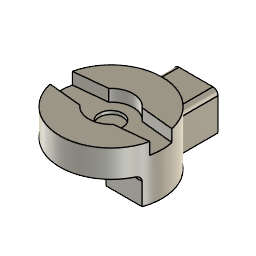
valve_coupler (Autodesk Fusion 360 design; units mm, degrees)
Autodesk Fusion 360 part; units mm, degrees
sketch "Sketch1" plane through (0, 0, 0) normal (0, 0, 1) x (1, 0, 0)
  circle A0 centre (0, 0) radius 6.5
  line L0 (-15, 0) -> (15, 0) construction
  line L1 (0, 15) -> (0, -15) construction
  arc A1 (-14.6437, -3.25) -> (0, -15) centre (0, 0) ccw
  arc A2 (14.6437, -3.25) -> (14.6437, 3.25) centre (0, 0) ccw
  arc A3 (-14.6437, 3.25) -> (-14.6437, -3.25) centre (0, 0) ccw
  arc A4 (0, 15) -> (-14.6437, 3.25) centre (0, 0) ccw
  arc A5 (0, -15) -> (14.6437, -3.25) centre (0, 0) ccw
  arc A6 (14.6437, 3.25) -> (0, 15) centre (0, 0) ccw
  line L2 (4.9181, 4.25) -> (4.9181, -4.25)
  line L3 (14.6437, 3.25) -> (14.6437, -3.25)
  line L4 (4.9181, -4.25) -> (14.6437, -3.25)
  line L5 (4.9181, 4.25) -> (14.6437, 3.25)
  line L6 (-14.6437, 3.25) -> (-14.6437, -3.25)
  line L7 (-4.9181, -4.25) -> (-14.6437, -3.25)
  line L8 (-4.9181, 4.25) -> (-4.9181, -4.25)
  line L9 (-4.9181, 4.25) -> (-14.6437, 3.25)
  circle A7 centre (0, 0) radius 3.5
  dimension "d1" = 30
  dimension "d2" = 13
  dimension "d5" = 6.5
  dimension "d6" = 8.5
  dimension "d25" = 7
  constraint coincident A0.centre A1.centre
  constraint coincident L0.start A2
  constraint coincident L0.end A2
  constraint horizontal L0
  constraint horizontal A0.centre L0.start
  constraint perpendicular L0 L1
  constraint vertical A0.centre L1.end
  constraint concentric A1 A2
  constraint concentric A2 A3
  constraint concentric A2 A4
  constraint concentric A2 A5
  constraint concentric A2 A6
  constraint coincident A0 L2.start
  constraint coincident A0 L2.end
  constraint perpendicular L0 L2
  constraint perpendicular L0 L3
  constraint symmetric A2.end L1 A3.start
  constraint symmetric A2.start L1 A1.start
  constraint symmetric L1 L2.start L8.start
  constraint symmetric L1 L2.end L7.start
  constraint concentric A4 A7
  measures "d1" diameter of A2
  measures "d2" diameter of A0
  measures "d5" vertical distance of A2.end A2.start
  measures "d6" vertical distance of L2.start L2.end
  measures "d25" diameter of A7
extrude "Extrude1" add sketch "Sketch1" along normal blind 16 contours A0 L2 | A0 L3 L4 L5 | A0 L2 L8 | A0 A4 A6 L5 L9 | A0 A1 A5 L4 L7 | A0 L8 | A0 L6 L7 L9 | A2 L3 | A3 L6 | A7
extrude "Extrude2" cut sketch "Sketch1" against normal blind 3.5 from surface at 16 contours A0 L2 | A0 L3 L4 L5 | A0 L2 L8 | A0 L8 | A0 L6 L7 L9 | A2 L3 | A3 L6 | A7
sketch "Sketch2" plane through (0, 0, 0) normal (0, 0, 1) x (1, 0, 0)
  arc A0 (-14.6437, -3.25) -> (0, -15) centre (0, 0) ccw
  arc A1 (0, -15) -> (14.6437, -3.25) centre (0, 0) ccw
  arc A2 (14.6437, -3.25) -> (14.6437, 3.25) centre (0, 0) ccw
  arc A3 (14.6437, 3.25) -> (0, 15) centre (0, 0) ccw
  arc A4 (0, 15) -> (-14.6437, 3.25) centre (0, 0) ccw
  arc A5 (-14.6437, 3.25) -> (-14.6437, -3.25) centre (0, 0) ccw
  line L0 (3.5, 15) -> (-3.5, 15)
  line L1 (-3.5, 15) -> (-3.5, -15)
  line L2 (-3.5, -15) -> (3.5, -15)
  line L3 (3.5, -15) -> (3.5, 15)
  line L4 (3.5, 15) -> (-3.5, -15) construction
  line L5 (-3.5, 15) -> (3.5, -15) construction
  dimension "d29" = 7
  dimension "d30" = 30
  constraint horizontal L0
  constraint perpendicular L0 L1
  constraint parallel L0 L2
  constraint parallel L1 L3
  constraint coincident L4 A0.centre
  constraint coincident L5 A0.centre
  constraint coincident A0.centre A1.centre
  measures "d29" distance of L1.end L2.end
  measures "d30" distance of L0.end L1.end
extrude "Extrude5" cut sketch "Sketch1" against normal blind 1 from surface at 12.5 contours A7
extrude "Extrude6" cut sketch "Sketch2" along normal blind 8 contours A0 A1 A3 A4 L1 L3
sketch "Sketch3" plane through (0, 0, 0) normal (0, 0, 1) x (1, 0, 0)
  arc A0 (0, 15) -> (-14.6437, 3.25) centre (0, 0) ccw construction
  arc A1 (-14.6437, 3.25) -> (-14.6437, -3.25) centre (0, 0) ccw construction
  arc A2 (-14.6437, -3.25) -> (0, -15) centre (0, 0) ccw construction
  arc A3 (0, -15) -> (14.6437, -3.25) centre (0, 0) ccw construction
  arc A4 (14.6437, 3.25) -> (0, 15) centre (0, 0) ccw construction
  arc A5 (14.6437, -3.25) -> (14.6437, 3.25) centre (0, 0) ccw construction
  line L0 (15, -15) -> (15, -5)
  line L1 (15, -5) -> (-15, -5)
  line L2 (-15, -5) -> (-15, -15)
  line L3 (0, 15) -> (0, 10) construction
  line L4 (6.5, 10) -> (6.5, 25)
  line L5 (6.5, 25) -> (-6.5, 25)
  line L6 (-6.5, 25) -> (-6.5, 10)
  line L7 (-11.1803, 10) -> (-6.5, 10) construction
  line L8 (6.5, 10) -> (11.1803, 10) construction
  line L9 (-6.5, 10) -> (0, 10)
  line L10 (0, 10) -> (6.5, 10)
  line L11 (3.5, 15) -> (-3.5, 15) construction
  line L12 (3.5, -15) -> (3.5, 15)
  line L13 (-3.5, -15) -> (3.5, -15) construction
  line L14 (-3.5, 15) -> (-3.5, -15)
  line L15 (15, -15) -> (-15, -15)
  line L16 (-3.5, 15) -> (-3.5, 25)
  line L17 (3.5, 15) -> (3.5, 25)
  dimension "d38" = 10
  dimension "d39" = 30
  dimension "d40" = 5
  dimension "d41" = 15
  dimension "d42" = 13
  dimension "d43" = 6.5
  dimension "d46" = 15
  constraint perpendicular L0 L1
  constraint perpendicular L1 L2
  constraint coincident A0.start A4.end
  constraint vertical L3
  constraint coincident A0 L7.start
  constraint coincident A4 L8.end
  constraint perpendicular L3 L7
  constraint horizontal L3.end L7.start
  constraint coincident L4.start L7
  constraint perpendicular L4 L7
  constraint perpendicular L4 L5
  constraint perpendicular L6 L7
  constraint perpendicular L4 L8
  constraint perpendicular L2 L15
  constraint tangent A2 L15
  constraint coincident A2.end L15
  constraint coincident L11.end L14.start
  constraint coincident L5 L16.end
  constraint perpendicular L5 L16
  constraint coincident L11.start L12.end
  constraint coincident L5 L17.end
  constraint perpendicular L5 L17
  measures "d38" distance of L0.start L0.end
  measures "d39" distance of L0.end L1.end
  measures "d40" distance of A0.start L3.end
  measures "d41" distance of L4.start L4.end
  measures "d42" distance of L4.end L5.end
  measures "d43" distance of L3 L6
  measures "d46" distance of L2.end L3
extrude "Extrude7 (1)" add sketch "Sketch3" along normal blind 11 contours L4 L5 L10 L12 L17 | L5 L9 L10 L12 L14 L16 L17 | L5 L6 L9 L14 L16
extrude "Extrude8" cut sketch "Sketch3" along normal blind 8 contours L0 L1 L12 L15 | L1 L12 L14 L15 | L1 L2 L14 L15 | L5 L9 L10 L12 L14 L16 L17
fillet "Fillet1" radius 1.5 2 edges at (6.5, 19.2593, 11) (-6.5, 19.2593, 11)
fillet "Fillet2" radius 1.5 2 edges at (8.8211, -5, 8) (-8.8211, -5, 8)
